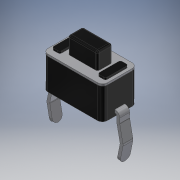
# Autodesk Inventor part: TACT-SWITCH-THT-3X6MM
Saved by Autodesk Inventor 2018.3 (Build 223284000, 284)
## iProperties
Created: 2020-10-19
Part Number: TACT-SWITCH-THT-3X6MM
Material: Genérico
Document SubType Name: Modeling
Designer: laguerre
Density: 8.47 g/cm^3
Appearance: Suave - Negro
Author: laguerre
Autodesk Inventor part; units mm, degrees
ref_plane "YZ Plane" through (0, 0, 0) normal (1, 0, 0) x (0, 1, 0)
ref_plane "XZ Plane" through (0, 0, 0) normal (0, 1, 0) x (-1, 0, 0)
ref_plane "XY Plane" through (0, 0, 0) normal (0, 0, 1) x (1, 0, 0)
sketch "Boceto39" plane through (0, 0, 0) normal (0, 0, 1) x (1, 0, 0)
  line L0 (-1.25, 3) -> (1.25, 3)
  line L1 (1.75, 2.5) -> (1.75, -2.5)
  line L2 (1.25, -3) -> (-1.25, -3)
  line L3 (-1.75, -2.5) -> (-1.75, 2.5)
  arc A0 (1.75, 2.5) -> (1.25, 3) centre (1.25, 2.5) ccw
  arc A1 (-1.25, 3) -> (-1.75, 2.5) centre (-1.25, 2.5) ccw
  arc A2 (-1.75, -2.5) -> (-1.25, -3) centre (-1.25, -2.5) ccw
  arc A3 (1.25, -3) -> (1.75, -2.5) centre (1.25, -2.5) ccw
  point P0 (0, 0)
  point P1 (-1.75, 3)
  point P2 (1.75, -3)
  point P3 (1.75, 3)
  point P4 (-1.75, -3)
  point P5 (0, 3)
  point P6 (1.75, 0)
  dimension "d373" = 3.5
  dimension "d376" = 0.5
  dimension "d437" = 6
  constraints: 8 end point, 8 point on circle, 8 point on line, 8 tangent, 4 centre point, 3 equal radius, 2 midpoint, 2 parallel, 1 horizontal, 1 horizontal alignment, 1 perpendicular, 1 vertical alignment
  measures "d373" distance of point (-1.75, 3) point (1.75, 3)
  measures "d376" radius of A0
  measures "d437" distance between parallel lines of L0 L2
extrude "Extrusión13" add sketch "Boceto39" along normal blind 3.1
sketch "Boceto40" plane through (0, 0, 3.1) normal (0, 0, 1) x (1, 0, 0)
  line L0 (1.25, 3) -> (-1.25, 3) projected
  arc A0 (-1.25, 3) -> (-1.75, 2.5) centre (-1.25, 2.5) ccw projected
  line L1 (-1.75, 2.5) -> (-1.75, -2.5) projected
  arc A1 (-1.75, -2.5) -> (-1.25, -3) centre (-1.25, -2.5) ccw projected
  line L2 (-1.25, -3) -> (1.25, -3) projected
  arc A2 (1.25, -3) -> (1.75, -2.5) centre (1.25, -2.5) ccw projected
  line L3 (1.75, -2.5) -> (1.75, 2.5) projected
  arc A3 (1.75, 2.5) -> (1.25, 3) centre (1.25, 2.5) ccw projected
  point P0 (0, 0)
extrude "Extrusión14" add sketch "Boceto40" along normal blind 0.2 separate body
sketch "Boceto43" plane through (0, 0, 0) normal (1, 0, 0) x (0, 1, 0)
  line L0 (0, 0) -> (0, -3.6276) construction
  line L1 (3, 0) -> (3, 3.1) construction
  line L2 (3, 0.6) -> (3, 0.6)
  line L3 (2.5, 3.3) -> (-2.5, 3.3) projected
  line L4 (2.5, 0) -> (-2.5, 0) projected
  line L5 (3.5, 0.1) -> (3.5, -0.3796)
  line L6 (3.5041, -0.42) -> (3.8297, -2.0012)
  line L7 (3.8304, -2.199) -> (3.4943, -3.9)
  line L8 (3.4943, -3.9) -> (3.2, -3.8418)
  line L9 (3.2, -3.8418) -> (3.5361, -2.1408)
  line L10 (3.5358, -2.0617) -> (3.2103, -0.4805)
  line L11 (3.2, -0.3796) -> (3.2, 0.1)
  line L12 (3, 0.3) -> (3, 0.3)
  line L13 (3, 0.3) -> (3, 0.6)
  arc A0 (3.2, 0.1) -> (3, 0.3) centre (3, 0.1) ccw
  arc A1 (3.5, -0.3796) -> (3.5041, -0.42) centre (3.7, -0.3796) ccw
  arc A2 (3.5361, -2.1408) -> (3.5358, -2.0617) centre (3.3399, -2.102) ccw
  arc A3 (3.5, 0.1) -> (3, 0.6) centre (3, 0.1) ccw
  arc A4 (3.2, -0.3796) -> (3.2103, -0.4805) centre (3.7, -0.3796) ccw
  arc A5 (3.8304, -2.199) -> (3.8297, -2.0012) centre (3.3399, -2.102) ccw
  point P0 (3.5, 0.6)
  point P1 (3.5, -0.4)
  point P2 (3.85, -2.1)
  point P3 (3.2, -0.4306)
  dimension "d399" = 2.7
  dimension "d426" = 0.3
  dimension "d427" = 0.3
  dimension "d428" = 0.3
  dimension "d429" = 0.3
  dimension "d430" = 3.85
  dimension "d431" = 3.2
  dimension "d432" = 3.9
  dimension "d433" = 1.8
  dimension "d434" = 1
  dimension "d435" = 0.2
  dimension "d436" = 0.5
  constraints: 22 end point, 12 point on circle, 12 tangent, 10 point on line, 6 centre point, 4 equal radius, 3 perpendicular, 2 parallel, 2 vertical, 1 collinear, 1 vertical alignment
  measures "d399" distance between parallel lines of L2 L3
  measures "d426" distance between parallel lines of L2 L12
  measures "d427" distance between parallel lines of L5 L11
  measures "d428" distance between parallel lines of L6 L10
  measures "d429" distance between parallel lines of L7 L9
  measures "d430" distance from line of point (3.85, -2.1) L0
  measures "d431" distance between parallel lines of L0 L11
  measures "d432" distance from line of L7.end L4
  measures "d433" vertical distance of point (3.85, -2.1) L7.end
  measures "d434" distance from line of L2 point (3.5, -0.4)
  measures "d435" radius of A0
  measures "d436" radius of A3
extrude "Extrusión15" add sketch "Boceto43" along normal mid plane 1 separate body
fillet "Empalme44" radius 0.5 2 edges at (0.5, 3.3472, -3.8709) (-0.5, 3.3472, -3.8709)
mirror "Simetría1" about plane through (0, 0, 0) normal (0, 1, 0) of "Extrusión15", "Empalme44" bodies 3
sketch "Boceto49" plane through (0, 0, 3.3) normal (0, 0, 1) x (1, 0, 0)
  line L0 (0.95, -2.7) -> (-0.95, -2.7)
  line L1 (-1.15, -2.5) -> (-1.15, -2.1)
  line L2 (-0.95, -1.9) -> (0.95, -1.9)
  line L3 (1.15, -2.1) -> (1.15, -2.5)
  line L4 (0.95, 1.9) -> (-0.95, 1.9)
  line L5 (-1.15, 2.1) -> (-1.15, 2.5)
  line L6 (-0.95, 2.7) -> (0.95, 2.7)
  line L7 (1.15, 2.5) -> (1.15, 2.1)
  arc A0 (0.95, -2.7) -> (1.15, -2.5) centre (0.95, -2.5) ccw
  arc A1 (1.15, -2.1) -> (0.95, -1.9) centre (0.95, -2.1) ccw
  arc A2 (-0.95, -1.9) -> (-1.15, -2.1) centre (-0.95, -2.1) ccw
  arc A3 (-1.15, -2.5) -> (-0.95, -2.7) centre (-0.95, -2.5) ccw
  arc A4 (-1.15, 2.1) -> (-0.95, 1.9) centre (-0.95, 2.1) ccw
  arc A5 (-0.95, 2.7) -> (-1.15, 2.5) centre (-0.95, 2.5) ccw
  arc A6 (1.15, 2.5) -> (0.95, 2.7) centre (0.95, 2.5) ccw
  arc A7 (0.95, 1.9) -> (1.15, 2.1) centre (0.95, 2.1) ccw
  line L8 (-1.15, 2.3) -> (1.15, 2.3) construction
  line L9 (-1.15, -2.3) -> (1.15, -2.3) construction
  line L10 (0.1537, -1.5) -> (-0.1537, -1.5) construction
  line L11 (-0.1537, -1.5) -> (-0.1537, 1.5) construction
  line L12 (-0.1537, 1.5) -> (0.1537, 1.5) construction
  line L13 (0.1537, 1.5) -> (0.1537, -1.5) construction
  point P0 (0, 0)
  point P1 (1.15, 1.9)
  point P2 (0, -2.7)
  point P3 (0, 1.9)
  point P4 (0, -1.5)
  point P5 (0.1537, 0)
  dimension "d438" = 0.8
  dimension "d439" = 0.2
  dimension "d441" = 2.3
  dimension "d442" = 2.3
  dimension "d443" = 3
  dimension "d444" = 2.3
  constraints: 28 end point, 16 point on circle, 16 tangent, 8 centre point, 8 midpoint, 7 equal radius, 6 parallel, 3 horizontal, 3 perpendicular, 3 point on line, 3 vertical alignment, 1 collinear, 1 horizontal alignment
  measures "d438" distance between parallel lines of L2 L0
  measures "d439" radius of A0
  measures "d441" distance from line of L9 point (0, 0)
  measures "d442" distance from line of point (0, 0) L8
  measures "d443" distance of L12.end L10.start
  measures "d444" distance of L9.start L9.end
extrude "Extrusión19" add sketch "Boceto49" along normal blind 0.2 bodies 2
sketch "Boceto50" plane through (0, 0, 0) normal (1, 0, 0) x (0, 1, 0)
  line L0 (-2.5, 3.3) -> (2.5, 3.3) projected
  line L1 (-1.5, 3.3) -> (1.5, 3.3)
  line L2 (1.5, 3.3) -> (1.5, 5)
  line L3 (1.5, 5) -> (-1.5, 5)
  line L4 (-1.5, 5) -> (-1.5, 3.3)
  line L5 (2.5, 0) -> (-2.5, 0) projected
  point P0 (0, 0)
  point P1 (0, 5)
  dimension "d447" = 5
  dimension "d448" = 3
  constraints: 8 end point, 2 parallel, 1 horizontal, 1 midpoint, 1 perpendicular, 1 point on line, 1 vertical alignment
  measures "d447" distance between parallel lines of L5 L3
  measures "d448" distance of L2.end L3.end
extrude "Extrusión20" add sketch "Boceto50" along normal mid plane 1.5 bodies 2
fillet "Empalme45" radius 0.2 8 edges at (0.75, 0, 5) (0, -1.5, 5) (-0.75, 0, 5) (0, 1.5, 5) (0.75, 1.5, 4.15) (-0.75, 1.5, 4.15) (0.75, -1.5, 4.15) (-0.75, -1.5, 4.15)
